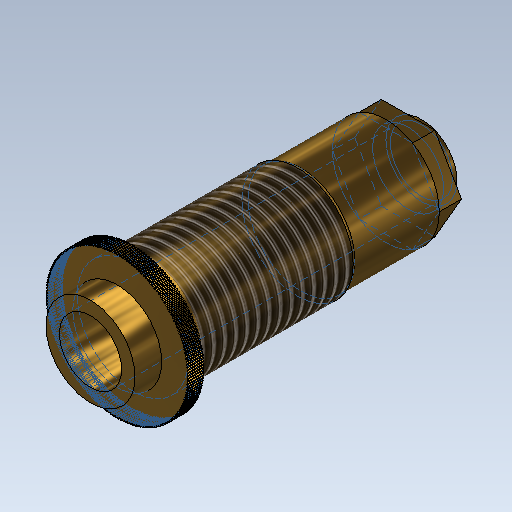
# Autodesk Inventor part: タミヤダンパー2
Saved by Autodesk Inventor 2020 (Build 240168000, 168)
## iProperties
Part Number: タミヤダンパー2
Material: 真鍮
Document SubType Name: Modeling
Designer: 雪村
Density: 8.49 g/cm^3
Appearance: 真鍮 - つや出し
Mass: 24.2679 g
Surface Area: 26.0167 cm^2
Volume: 2.85841 cm^3
Author: 雪村
Autodesk Inventor part; units mm, degrees
(part 1 of 2)
ref_plane "YZ Plane" through (0, 0, 0) normal (1, 0, 0) x (0, 1, 0)
ref_plane "XZ Plane" through (0, 0, 0) normal (0, 1, 0) x (-1, 0, 0)
ref_plane "XY Plane" through (0, 0, 0) normal (0, 0, 1) x (1, 0, 0)
sketch "スケッチ1" plane through (0, 0, 0) normal (0, 0, 1) x (1, 0, 0)
  circle A0 centre (0, 0) radius 5.5
  dimension "d0" = 11
  constraints: 1 centre point, 1 coincident
  measures "d0" diameter of A0
extrude "押し出し1" add sketch "スケッチ1" along normal blind 2.5
sketch "スケッチ2" plane through (0, 0, 2.5) normal (0, 0, 1) x (1, 0, 0)
  circle A0 centre (0, 0) radius 6
  dimension "d3" = 12
  constraints: 1 centre point, 1 coincident
  measures "d3" diameter of A0
extrude "押し出し2" add sketch "スケッチ2" along normal blind 9.5
sketch "スケッチ3" plane through (0, 0, 12) normal (0, 0, 1) x (1, 0, 0)
  circle A0 centre (0, 0) radius 6.25
  dimension "d6" = 12.5
  constraints: 1 centre point, 1 coincident
  measures "d6" diameter of A0
extrude "押し出し3" add sketch "スケッチ3" along normal blind 18.95
sketch "スケッチ4" plane through (0, 0, 30.95) normal (0, 0, 1) x (1, 0, 0)
  circle A0 centre (0, 0) radius 8
  dimension "d9" = 16
  constraints: 1 centre point, 1 coincident
  measures "d9" diameter of A0
extrude "押し出し4" add sketch "スケッチ4" along normal blind 1.75
sketch "スケッチ5" plane through (0, 0, 0) normal (0, 0, -1) x (-1, 0, 0)
  line L0 (-3, -5.1962) -> (-6, 0)
  line L1 (-6, 0) -> (-3, 5.1962)
  line L2 (-3, 5.1962) -> (3, 5.1962)
  line L3 (3, 5.1962) -> (6, 0)
  line L4 (6, 0) -> (3, -5.1962)
  line L5 (3, -5.1962) -> (-3, -5.1962)
  circle A0 centre (0, 0) radius 6 projected
  constraints: 12 end point, 1 coincident, 1 horizontal, 15 other
extrude "押し出し5" add sketch "スケッチ5" against normal blind 2.5 contours L0 L1 L2 L3 L4 L5
sketch "スケッチ6" plane through (0, 0, 0) normal (0, 0, -1) x (-1, 0, 0)
  arc A0 (3.5986, -4.1593) -> (5.4014, -1.0368) centre (0, 0) ccw projected
  line L0 (6, 0) -> (5.4014, -1.0368) projected
  line L1 (5.4014, 1.0368) -> (6, 0) projected
  arc A1 (5.4014, 1.0368) -> (3.5986, 4.1593) centre (0, 0) ccw projected
  line L2 (3, 5.1962) -> (3.5986, 4.1593) projected
  line L3 (1.8028, 5.1962) -> (3, 5.1962) projected
  arc A2 (1.8028, 5.1962) -> (-1.8028, 5.1962) centre (0, 0) ccw projected
  line L4 (-3, 5.1962) -> (-1.8028, 5.1962) projected
  line L5 (-3.5986, 4.1593) -> (-3, 5.1962) projected
  arc A3 (-3.5986, 4.1593) -> (-5.4014, 1.0368) centre (0, 0) ccw projected
  line L6 (-6, 0) -> (-5.4014, 1.0368) projected
  line L7 (-5.4014, -1.0368) -> (-6, 0) projected
  arc A4 (-5.4014, -1.0368) -> (-3.5986, -4.1593) centre (0, 0) ccw projected
  line L8 (-3, -5.1962) -> (-3.5986, -4.1593) projected
  line L9 (-1.8028, -5.1962) -> (-3, -5.1962) projected
  arc A5 (-1.8028, -5.1962) -> (1.8028, -5.1962) centre (0, 0) ccw projected
  line L10 (3, -5.1962) -> (1.8028, -5.1962) projected
  line L11 (3.5986, -4.1593) -> (3, -5.1962) projected
  line L12 (3, -5.1962) -> (-3, -5.1962)
  line L13 (-3, -5.1962) -> (-6, 0)
  line L14 (-6, 0) -> (-3, 5.1962)
  line L15 (-3, 5.1962) -> (3, 5.1962)
  line L16 (3, 5.1962) -> (6, 0)
  line L17 (6, 0) -> (3, -5.1962)
  constraints: 12 end point, 1 coincident, 13 other
extrude "押し出し6" cut sketch "スケッチ6" against normal blind 2.5 contours L17 A0 | A5 L12 | L16 A1 | A4 L13 | L15 A2 | A3 L14
sketch "スケッチ8" plane through (0, 0, 0) normal (0, 0, -1) x (-1, 0, 0)
  circle A0 centre (0, 0) radius 3.5
  dimension "d22" = 7
  constraints: 1 centre point, 1 coincident
  measures "d22" diameter of A0
extrude "押し出し7" cut sketch "スケッチ8" against normal through all
sketch "スケッチ9" plane through (0, 0, 32.7) normal (0, 0, 1) x (1, 0, 0)
  circle A0 centre (0, 0) radius 3.5 projected
  circle A1 centre (0, 0) radius 5
  dimension "d25" = 10
  constraints: 1 centre point, 1 coincident
  measures "d25" diameter of A1
extrude "押し出し8" add sketch "スケッチ9" along normal blind 3
sketch "スケッチ11" plane through (0, 0, 0) normal (0, 0, -1) x (-1, 0, 0)
  circle A0 centre (0, 0) radius 3.5 projected
  circle A1 centre (0, 0) radius 4
  dimension "d28" = 8
  constraints: 1 centre point, 1 coincident
  measures "d28" diameter of A1
extrude "押し出し9" add sketch "スケッチ11" along normal blind 1.5
sketch "スケッチ12" plane through (0, 0, 32.7) normal (0, 0, 1) x (1, 0, 0)
  arc A0 (0.0868, 7.9995) -> (-0.0868, 7.9995) centre (0, 0) ccw
  arc A1 (0.05, 7.8748) -> (-0.05, 7.8748) centre (0, 0) ccw
  line L0 (-0.05, 7.8748) -> (-0.0868, 7.9995)
  line L1 (0.05, 7.8748) -> (0.0868, 7.9995)
  line L2 (0, 7.875) -> (0, 0)
  line L3 (-0.5992, 7.8522) -> (-0.6446, 7.974)
  arc A2 (-0.4714, 7.9861) -> (-0.6446, 7.974) centre (0, 0) ccw
  line L4 (-0.4994, 7.8591) -> (-0.4714, 7.9861)
  arc A3 (-0.4994, 7.8591) -> (-0.5992, 7.8522) centre (0, 0) ccw
  line L5 (-1.1455, 7.7912) -> (-1.1993, 7.9096)
  arc A4 (-1.0274, 7.9338) -> (-1.1993, 7.9096) centre (0, 0) ccw
  line L6 (-1.0465, 7.8052) -> (-1.0274, 7.9338)
  arc A5 (-1.0465, 7.8052) -> (-1.1455, 7.7912) centre (0, 0) ccw
  line L7 (-1.6862, 7.6924) -> (-1.7481, 7.8067)
  arc A6 (-1.5783, 7.8428) -> (-1.7481, 7.8067) centre (0, 0) ccw
  line L8 (-1.5884, 7.7132) -> (-1.5783, 7.8428)
  arc A7 (-1.5884, 7.7132) -> (-1.6862, 7.6924) centre (0, 0) ccw
  line L9 (-2.2187, 7.556) -> (-2.2884, 7.6657)
  arc A8 (-2.1215, 7.7136) -> (-2.2884, 7.6657) centre (0, 0) ccw
  line L10 (-2.1225, 7.5836) -> (-2.1215, 7.7136)
  arc A9 (-2.1225, 7.5836) -> (-2.2187, 7.556) centre (0, 0) ccw
  line L11 (-2.7403, 7.3828) -> (-2.8175, 7.4874)
  arc A10 (-2.6545, 7.5468) -> (-2.8175, 7.4874) centre (0, 0) ccw
  line L12 (-2.6464, 7.417) -> (-2.6545, 7.5468)
  arc A11 (-2.6464, 7.417) -> (-2.7403, 7.3828) centre (0, 0) ccw
  line L13 (-3.2487, 7.1737) -> (-3.333, 7.2726)
  arc A12 (-3.1744, 7.3432) -> (-3.333, 7.2726) centre (0, 0) ccw
  line L14 (-3.1573, 7.2144) -> (-3.1744, 7.3432)
  arc A13 (-3.1573, 7.2144) -> (-3.2487, 7.1737) centre (0, 0) ccw
  line L15 (-3.7412, 6.9296) -> (-3.8322, 7.0224)
  arc A14 (-3.6789, 7.1039) -> (-3.8322, 7.0224) centre (0, 0) ccw
  line L16 (-3.6529, 6.9765) -> (-3.6789, 7.1039)
  arc A15 (-3.6529, 6.9765) -> (-3.7412, 6.9296) centre (0, 0) ccw
  line L17 (-4.2154, 6.6517) -> (-4.3127, 6.738)
  arc A16 (-4.1655, 6.83) -> (-4.3127, 6.738) centre (0, 0) ccw
  line L18 (-4.1306, 6.7047) -> (-4.1655, 6.83)
  arc A17 (-4.1306, 6.7047) -> (-4.2154, 6.6517) centre (0, 0) ccw
  line L19 (-4.6692, 6.3415) -> (-4.7722, 6.4207)
  arc A18 (-4.6318, 6.5228) -> (-4.7722, 6.4207) centre (0, 0) ccw
  line L20 (-4.5883, 6.4003) -> (-4.6318, 6.5228)
  arc A19 (-4.5883, 6.4003) -> (-4.6692, 6.3415) centre (0, 0) ccw
  line L21 (-5.1002, 6.0003) -> (-5.2085, 6.0722)
  arc A20 (-5.0755, 6.1838) -> (-5.2085, 6.0722) centre (0, 0) ccw
  line L22 (-5.0235, 6.0646) -> (-5.0755, 6.1838)
  arc A21 (-5.0235, 6.0646) -> (-5.1002, 6.0003) centre (0, 0) ccw
  line L23 (-5.5063, 5.63) -> (-5.6194, 5.6941)
  arc A22 (-5.4945, 5.8147) -> (-5.6194, 5.6941) centre (0, 0) ccw
  line L24 (-5.4344, 5.6994) -> (-5.4945, 5.8147)
  arc A23 (-5.4344, 5.6994) -> (-5.5063, 5.63) centre (0, 0) ccw
  line L25 (-5.8856, 5.2321) -> (-6.0029, 5.2882)
  arc A24 (-5.8867, 5.4172) -> (-6.0029, 5.2882) centre (0, 0) ccw
  line L26 (-5.8187, 5.3065) -> (-5.8867, 5.4172)
  arc A25 (-5.8187, 5.3065) -> (-5.8856, 5.2321) centre (0, 0) ccw
  line L27 (-6.2362, 4.8088) -> (-6.3571, 4.8566)
  arc A26 (-6.2503, 4.9934) -> (-6.3571, 4.8566) centre (0, 0) ccw
  line L28 (-6.1747, 4.8876) -> (-6.2503, 4.9934)
  arc A27 (-6.1747, 4.8876) -> (-6.2362, 4.8088) centre (0, 0) ccw
  line L29 (-6.5565, 4.3621) -> (-6.6804, 4.4013)
  arc A28 (-6.5834, 4.5452) -> (-6.6804, 4.4013) centre (0, 0) ccw
  line L30 (-6.5006, 4.445) -> (-6.5834, 4.5452)
  arc A29 (-6.5006, 4.445) -> (-6.5565, 4.3621) centre (0, 0) ccw
  line L31 (-6.8448, 3.8941) -> (-6.9712, 3.9246)
  arc A30 (-6.8844, 4.0749) -> (-6.9712, 3.9246) centre (0, 0) ccw
  line L32 (-6.7948, 3.9807) -> (-6.8844, 4.0749)
  arc A31 (-6.7948, 3.9807) -> (-6.8448, 3.8941) centre (0, 0) ccw
  line L33 (-7.0998, 3.4072) -> (-7.228, 3.4288)
  arc A32 (-7.1519, 3.5848) -> (-7.228, 3.4288) centre (0, 0) ccw
  line L34 (-7.0559, 3.497) -> (-7.1519, 3.5848)
  arc A33 (-7.0559, 3.497) -> (-7.0998, 3.4072) centre (0, 0) ccw
  line L35 (-7.3202, 2.9036) -> (-7.4495, 2.9162)
  arc A34 (-7.3845, 3.0771) -> (-7.4495, 2.9162) centre (0, 0) ccw
  line L36 (-7.2827, 2.9963) -> (-7.3845, 3.0771)
  arc A35 (-7.2827, 2.9963) -> (-7.3202, 2.9036) centre (0, 0) ccw
  line L37 (-7.5049, 2.3859) -> (-7.6348, 2.3895)
  arc A36 (-7.5812, 2.5545) -> (-7.6348, 2.3895) centre (0, 0) ccw
  line L38 (-7.474, 2.481) -> (-7.5812, 2.5545)
  arc A37 (-7.474, 2.481) -> (-7.5049, 2.3859) centre (0, 0) ccw
  line L39 (-7.653, 1.8566) -> (-7.7829, 1.8511)
  arc A38 (-7.7409, 2.0195) -> (-7.7829, 1.8511) centre (0, 0) ccw
  line L40 (-7.6288, 1.9536) -> (-7.7409, 2.0195)
  arc A39 (-7.6288, 1.9536) -> (-7.653, 1.8566) centre (0, 0) ccw
  line L41 (-7.7639, 1.3182) -> (-7.8931, 1.3036)
  arc A40 (-7.8629, 1.4746) -> (-7.8931, 1.3036) centre (0, 0) ccw
  line L42 (-7.7465, 1.4167) -> (-7.8629, 1.4746)
  arc A41 (-7.7465, 1.4167) -> (-7.7639, 1.3182) centre (0, 0) ccw
  line L43 (-7.8369, 0.7734) -> (-7.9648, 0.7499)
  arc A42 (-7.9466, 0.9225) -> (-7.9648, 0.7499) centre (0, 0) ccw
  line L44 (-7.8265, 0.8729) -> (-7.9466, 0.9225)
  arc A43 (-7.8265, 0.8729) -> (-7.8369, 0.7734) centre (0, 0) ccw
  line L45 (-7.8718, 0.2249) -> (-7.9977, 0.1925)
  arc A44 (-7.9916, 0.3659) -> (-7.9977, 0.1925) centre (0, 0) ccw
  line L46 (-7.8683, 0.3248) -> (-7.9916, 0.3659)
  arc A45 (-7.8683, 0.3248) -> (-7.8718, 0.2249) centre (0, 0) ccw
  line L47 (-7.8683, -0.3248) -> (-7.9916, -0.3659)
  arc A46 (-7.9977, -0.1925) -> (-7.9916, -0.3659) centre (0, 0) ccw
  line L48 (-7.8718, -0.2249) -> (-7.9977, -0.1925)
  arc A47 (-7.8718, -0.2249) -> (-7.8683, -0.3248) centre (0, 0) ccw
  line L49 (-7.8265, -0.8729) -> (-7.9466, -0.9225)
  arc A48 (-7.9648, -0.7499) -> (-7.9466, -0.9225) centre (0, 0) ccw
  line L50 (-7.8369, -0.7734) -> (-7.9648, -0.7499)
  arc A49 (-7.8369, -0.7734) -> (-7.8265, -0.8729) centre (0, 0) ccw
  line L51 (-7.7465, -1.4167) -> (-7.8629, -1.4746)
  arc A50 (-7.8931, -1.3036) -> (-7.8629, -1.4746) centre (0, 0) ccw
  line L52 (-7.7639, -1.3182) -> (-7.8931, -1.3036)
  arc A51 (-7.7639, -1.3182) -> (-7.7465, -1.4167) centre (0, 0) ccw
  line L53 (-7.6288, -1.9536) -> (-7.7409, -2.0195)
  arc A52 (-7.7829, -1.8511) -> (-7.7409, -2.0195) centre (0, 0) ccw
  line L54 (-7.653, -1.8566) -> (-7.7829, -1.8511)
  arc A53 (-7.653, -1.8566) -> (-7.6288, -1.9536) centre (0, 0) ccw
  line L55 (-7.474, -2.481) -> (-7.5812, -2.5545)
  arc A54 (-7.6348, -2.3895) -> (-7.5812, -2.5545) centre (0, 0) ccw
  line L56 (-7.5049, -2.3859) -> (-7.6348, -2.3895)
  arc A55 (-7.5049, -2.3859) -> (-7.474, -2.481) centre (0, 0) ccw
  line L57 (-7.2827, -2.9963) -> (-7.3845, -3.0771)
  arc A56 (-7.4495, -2.9162) -> (-7.3845, -3.0771) centre (0, 0) ccw
  line L58 (-7.3202, -2.9036) -> (-7.4495, -2.9162)
  arc A57 (-7.3202, -2.9036) -> (-7.2827, -2.9963) centre (0, 0) ccw
  line L59 (-7.0559, -3.497) -> (-7.1519, -3.5848)
  arc A58 (-7.228, -3.4288) -> (-7.1519, -3.5848) centre (0, 0) ccw
  line L60 (-7.0998, -3.4072) -> (-7.228, -3.4288)
  arc A59 (-7.0998, -3.4072) -> (-7.0559, -3.497) centre (0, 0) ccw
  line L61 (-6.7948, -3.9807) -> (-6.8844, -4.0749)
  arc A60 (-6.9712, -3.9246) -> (-6.8844, -4.0749) centre (0, 0) ccw
  line L62 (-6.8448, -3.8941) -> (-6.9712, -3.9246)
  arc A61 (-6.8448, -3.8941) -> (-6.7948, -3.9807) centre (0, 0) ccw
  line L63 (-6.5006, -4.445) -> (-6.5834, -4.5452)
  arc A62 (-6.6804, -4.4013) -> (-6.5834, -4.5452) centre (0, 0) ccw
  line L64 (-6.5565, -4.3621) -> (-6.6804, -4.4013)
  arc A63 (-6.5565, -4.3621) -> (-6.5006, -4.445) centre (0, 0) ccw
  line L65 (-6.1747, -4.8876) -> (-6.2503, -4.9934)
  arc A64 (-6.3571, -4.8566) -> (-6.2503, -4.9934) centre (0, 0) ccw
  line L66 (-6.2362, -4.8088) -> (-6.3571, -4.8566)
  arc A65 (-6.2362, -4.8088) -> (-6.1747, -4.8876) centre (0, 0) ccw
  line L67 (-5.8187, -5.3065) -> (-5.8867, -5.4172)
  arc A66 (-6.0029, -5.2882) -> (-5.8867, -5.4172) centre (0, 0) ccw
  line L68 (-5.8856, -5.2321) -> (-6.0029, -5.2882)
  arc A67 (-5.8856, -5.2321) -> (-5.8187, -5.3065) centre (0, 0) ccw
  line L69 (-5.4344, -5.6994) -> (-5.4945, -5.8147)
  arc A68 (-5.6194, -5.6941) -> (-5.4945, -5.8147) centre (0, 0) ccw
  line L70 (-5.5063, -5.63) -> (-5.6194, -5.6941)
  arc A69 (-5.5063, -5.63) -> (-5.4344, -5.6994) centre (0, 0) ccw
  line L71 (-5.0235, -6.0646) -> (-5.0755, -6.1838)
  arc A70 (-5.2085, -6.0722) -> (-5.0755, -6.1838) centre (0, 0) ccw
  line L72 (-5.1002, -6.0003) -> (-5.2085, -6.0722)
  arc A71 (-5.1002, -6.0003) -> (-5.0235, -6.0646) centre (0, 0) ccw
  line L73 (-4.5883, -6.4003) -> (-4.6318, -6.5228)
  arc A72 (-4.7722, -6.4207) -> (-4.6318, -6.5228) centre (0, 0) ccw
  line L74 (-4.6692, -6.3415) -> (-4.7722, -6.4207)
  arc A73 (-4.6692, -6.3415) -> (-4.5883, -6.4003) centre (0, 0) ccw
  line L75 (-4.1306, -6.7047) -> (-4.1655, -6.83)
  arc A74 (-4.3127, -6.738) -> (-4.1655, -6.83) centre (0, 0) ccw
  line L76 (-4.2154, -6.6517) -> (-4.3127, -6.738)
  arc A75 (-4.2154, -6.6517) -> (-4.1306, -6.7047) centre (0, 0) ccw
  line L77 (-3.6529, -6.9765) -> (-3.6789, -7.1039)
  arc A76 (-3.8322, -7.0224) -> (-3.6789, -7.1039) centre (0, 0) ccw
  line L78 (-3.7412, -6.9296) -> (-3.8322, -7.0224)
  arc A77 (-3.7412, -6.9296) -> (-3.6529, -6.9765) centre (0, 0) ccw
  line L79 (-3.1573, -7.2144) -> (-3.1744, -7.3432)
  arc A78 (-3.333, -7.2726) -> (-3.1744, -7.3432) centre (0, 0) ccw
  line L80 (-3.2487, -7.1737) -> (-3.333, -7.2726)
  arc A79 (-3.2487, -7.1737) -> (-3.1573, -7.2144) centre (0, 0) ccw
  line L81 (-2.6464, -7.417) -> (-2.6545, -7.5468)
  arc A80 (-2.8175, -7.4874) -> (-2.6545, -7.5468) centre (0, 0) ccw
  line L82 (-2.7403, -7.3828) -> (-2.8175, -7.4874)
  arc A81 (-2.7403, -7.3828) -> (-2.6464, -7.417) centre (0, 0) ccw
  line L83 (-2.1225, -7.5836) -> (-2.1215, -7.7136)
  arc A82 (-2.2884, -7.6657) -> (-2.1215, -7.7136) centre (0, 0) ccw
  line L84 (-2.2187, -7.556) -> (-2.2884, -7.6657)
  arc A83 (-2.2187, -7.556) -> (-2.1225, -7.5836) centre (0, 0) ccw
  line L85 (-1.5884, -7.7132) -> (-1.5783, -7.8428)
  arc A84 (-1.7481, -7.8067) -> (-1.5783, -7.8428) centre (0, 0) ccw
  line L86 (-1.6862, -7.6924) -> (-1.7481, -7.8067)
  arc A85 (-1.6862, -7.6924) -> (-1.5884, -7.7132) centre (0, 0) ccw
  line L87 (-1.0465, -7.8052) -> (-1.0274, -7.9338)
  arc A86 (-1.1993, -7.9096) -> (-1.0274, -7.9338) centre (0, 0) ccw
  line L88 (-1.1455, -7.7912) -> (-1.1993, -7.9096)
  arc A87 (-1.1455, -7.7912) -> (-1.0465, -7.8052) centre (0, 0) ccw
  line L89 (-0.4994, -7.8591) -> (-0.4714, -7.9861)
  arc A88 (-0.6446, -7.974) -> (-0.4714, -7.9861) centre (0, 0) ccw
  line L90 (-0.5992, -7.8522) -> (-0.6446, -7.974)
  arc A89 (-0.5992, -7.8522) -> (-0.4994, -7.8591) centre (0, 0) ccw
  line L91 (0.05, -7.8748) -> (0.0868, -7.9995)
  arc A90 (-0.0868, -7.9995) -> (0.0868, -7.9995) centre (0, 0) ccw
  line L92 (-0.05, -7.8748) -> (-0.0868, -7.9995)
  arc A91 (-0.05, -7.8748) -> (0.05, -7.8748) centre (0, 0) ccw
  line L93 (0.5992, -7.8522) -> (0.6446, -7.974)
  arc A92 (0.4714, -7.9861) -> (0.6446, -7.974) centre (0, 0) ccw
  line L94 (0.4994, -7.8591) -> (0.4714, -7.9861)
  arc A93 (0.4994, -7.8591) -> (0.5992, -7.8522) centre (0, 0) ccw
  line L95 (1.1455, -7.7912) -> (1.1993, -7.9096)
  arc A94 (1.0274, -7.9338) -> (1.1993, -7.9096) centre (0, 0) ccw
  line L96 (1.0465, -7.8052) -> (1.0274, -7.9338)
  arc A95 (1.0465, -7.8052) -> (1.1455, -7.7912) centre (0, 0) ccw
  line L97 (1.6862, -7.6924) -> (1.7481, -7.8067)
  arc A96 (1.5783, -7.8428) -> (1.7481, -7.8067) centre (0, 0) ccw
  line L98 (1.5884, -7.7132) -> (1.5783, -7.8428)
  arc A97 (1.5884, -7.7132) -> (1.6862, -7.6924) centre (0, 0) ccw
  line L99 (2.2187, -7.556) -> (2.2884, -7.6657)
  arc A98 (2.1215, -7.7136) -> (2.2884, -7.6657) centre (0, 0) ccw
  line L100 (2.1225, -7.5836) -> (2.1215, -7.7136)
  arc A99 (2.1225, -7.5836) -> (2.2187, -7.556) centre (0, 0) ccw
  line L101 (2.7403, -7.3828) -> (2.8175, -7.4874)
  arc A100 (2.6545, -7.5468) -> (2.8175, -7.4874) centre (0, 0) ccw
  line L102 (2.6464, -7.417) -> (2.6545, -7.5468)
  arc A101 (2.6464, -7.417) -> (2.7403, -7.3828) centre (0, 0) ccw
  line L103 (3.2487, -7.1737) -> (3.333, -7.2726)
  arc A102 (3.1744, -7.3432) -> (3.333, -7.2726) centre (0, 0) ccw
  line L104 (3.1573, -7.2144) -> (3.1744, -7.3432)
  arc A103 (3.1573, -7.2144) -> (3.2487, -7.1737) centre (0, 0) ccw
  line L105 (3.7412, -6.9296) -> (3.8322, -7.0224)
  arc A104 (3.6789, -7.1039) -> (3.8322, -7.0224) centre (0, 0) ccw
  line L106 (3.6529, -6.9765) -> (3.6789, -7.1039)
  arc A105 (3.6529, -6.9765) -> (3.7412, -6.9296) centre (0, 0) ccw
  line L107 (4.2154, -6.6517) -> (4.3127, -6.738)
  arc A106 (4.1655, -6.83) -> (4.3127, -6.738) centre (0, 0) ccw
  line L108 (4.1306, -6.7047) -> (4.1655, -6.83)
  arc A107 (4.1306, -6.7047) -> (4.2154, -6.6517) centre (0, 0) ccw
  line L109 (4.6692, -6.3415) -> (4.7722, -6.4207)
  arc A108 (4.6318, -6.5228) -> (4.7722, -6.4207) centre (0, 0) ccw
  line L110 (4.5883, -6.4003) -> (4.6318, -6.5228)
  arc A109 (4.5883, -6.4003) -> (4.6692, -6.3415) centre (0, 0) ccw
  line L111 (5.1002, -6.0003) -> (5.2085, -6.0722)
  arc A110 (5.0755, -6.1838) -> (5.2085, -6.0722) centre (0, 0) ccw
  line L112 (5.0235, -6.0646) -> (5.0755, -6.1838)
  arc A111 (5.0235, -6.0646) -> (5.1002, -6.0003) centre (0, 0) ccw
  line L113 (5.5063, -5.63) -> (5.6194, -5.6941)
  arc A112 (5.4945, -5.8147) -> (5.6194, -5.6941) centre (0, 0) ccw
  line L114 (5.4344, -5.6994) -> (5.4945, -5.8147)
  arc A113 (5.4344, -5.6994) -> (5.5063, -5.63) centre (0, 0) ccw
  line L115 (5.8856, -5.2321) -> (6.0029, -5.2882)
  arc A114 (5.8867, -5.4172) -> (6.0029, -5.2882) centre (0, 0) ccw
  line L116 (5.8187, -5.3065) -> (5.8867, -5.4172)
  arc A115 (5.8187, -5.3065) -> (5.8856, -5.2321) centre (0, 0) ccw
  line L117 (6.2362, -4.8088) -> (6.3571, -4.8566)
  arc A116 (6.2503, -4.9934) -> (6.3571, -4.8566) centre (0, 0) ccw
  line L118 (6.1747, -4.8876) -> (6.2503, -4.9934)
  arc A117 (6.1747, -4.8876) -> (6.2362, -4.8088) centre (0, 0) ccw
  line L119 (6.5565, -4.3621) -> (6.6804, -4.4013)
  arc A118 (6.5834, -4.5452) -> (6.6804, -4.4013) centre (0, 0) ccw
  line L120 (6.5006, -4.445) -> (6.5834, -4.5452)
  arc A119 (6.5006, -4.445) -> (6.5565, -4.3621) centre (0, 0) ccw
  line L121 (6.8448, -3.8941) -> (6.9712, -3.9246)
  arc A120 (6.8844, -4.0749) -> (6.9712, -3.9246) centre (0, 0) ccw
  line L122 (6.7948, -3.9807) -> (6.8844, -4.0749)
  arc A121 (6.7948, -3.9807) -> (6.8448, -3.8941) centre (0, 0) ccw
  line L123 (7.0998, -3.4072) -> (7.228, -3.4288)
  arc A122 (7.1519, -3.5848) -> (7.228, -3.4288) centre (0, 0) ccw
  line L124 (7.0559, -3.497) -> (7.1519, -3.5848)
  arc A123 (7.0559, -3.497) -> (7.0998, -3.4072) centre (0, 0) ccw
  line L125 (7.3202, -2.9036) -> (7.4495, -2.9162)
  arc A124 (7.3845, -3.0771) -> (7.4495, -2.9162) centre (0, 0) ccw
  line L126 (7.2827, -2.9963) -> (7.3845, -3.0771)
  arc A125 (7.2827, -2.9963) -> (7.3202, -2.9036) centre (0, 0) ccw
  line L127 (7.5049, -2.3859) -> (7.6348, -2.3895)
  arc A126 (7.5812, -2.5545) -> (7.6348, -2.3895) centre (0, 0) ccw
  line L128 (7.474, -2.481) -> (7.5812, -2.5545)
  arc A127 (7.474, -2.481) -> (7.5049, -2.3859) centre (0, 0) ccw
  line L129 (7.653, -1.8566) -> (7.7829, -1.8511)
  arc A128 (7.7409, -2.0195) -> (7.7829, -1.8511) centre (0, 0) ccw
  line L130 (7.6288, -1.9536) -> (7.7409, -2.0195)
  arc A129 (7.6288, -1.9536) -> (7.653, -1.8566) centre (0, 0) ccw
  line L131 (7.7639, -1.3182) -> (7.8931, -1.3036)
  arc A130 (7.8629, -1.4746) -> (7.8931, -1.3036) centre (0, 0) ccw
  line L132 (7.7465, -1.4167) -> (7.8629, -1.4746)
  arc A131 (7.7465, -1.4167) -> (7.7639, -1.3182) centre (0, 0) ccw
  line L133 (7.8369, -0.7734) -> (7.9648, -0.7499)
  arc A132 (7.9466, -0.9225) -> (7.9648, -0.7499) centre (0, 0) ccw
  line L134 (7.8265, -0.8729) -> (7.9466, -0.9225)
  arc A133 (7.8265, -0.8729) -> (7.8369, -0.7734) centre (0, 0) ccw
  line L135 (7.8718, -0.2249) -> (7.9977, -0.1925)
  arc A134 (7.9916, -0.3659) -> (7.9977, -0.1925) centre (0, 0) ccw
  line L136 (7.8683, -0.3248) -> (7.9916, -0.3659)
  arc A135 (7.8683, -0.3248) -> (7.8718, -0.2249) centre (0, 0) ccw
  line L137 (7.8683, 0.3248) -> (7.9916, 0.3659)
  arc A136 (7.9977, 0.1925) -> (7.9916, 0.3659) centre (0, 0) ccw
  line L138 (7.8718, 0.2249) -> (7.9977, 0.1925)
  arc A137 (7.8718, 0.2249) -> (7.8683, 0.3248) centre (0, 0) ccw
  line L139 (7.8265, 0.8729) -> (7.9466, 0.9225)
  arc A138 (7.9648, 0.7499) -> (7.9466, 0.9225) centre (0, 0) ccw
  line L140 (7.8369, 0.7734) -> (7.9648, 0.7499)
  arc A139 (7.8369, 0.7734) -> (7.8265, 0.8729) centre (0, 0) ccw
  line L141 (7.7465, 1.4167) -> (7.8629, 1.4746)
  arc A140 (7.8931, 1.3036) -> (7.8629, 1.4746) centre (0, 0) ccw
  line L142 (7.7639, 1.3182) -> (7.8931, 1.3036)
  arc A141 (7.7639, 1.3182) -> (7.7465, 1.4167) centre (0, 0) ccw
  line L143 (7.6288, 1.9536) -> (7.7409, 2.0195)
  arc A142 (7.7829, 1.8511) -> (7.7409, 2.0195) centre (0, 0) ccw
  line L144 (7.653, 1.8566) -> (7.7829, 1.8511)
  arc A143 (7.653, 1.8566) -> (7.6288, 1.9536) centre (0, 0) ccw
  line L145 (7.474, 2.481) -> (7.5812, 2.5545)
  arc A144 (7.6348, 2.3895) -> (7.5812, 2.5545) centre (0, 0) ccw
  line L146 (7.5049, 2.3859) -> (7.6348, 2.3895)
  arc A145 (7.5049, 2.3859) -> (7.474, 2.481) centre (0, 0) ccw
  line L147 (7.2827, 2.9963) -> (7.3845, 3.0771)
  arc A146 (7.4495, 2.9162) -> (7.3845, 3.0771) centre (0, 0) ccw
  line L148 (7.3202, 2.9036) -> (7.4495, 2.9162)
  arc A147 (7.3202, 2.9036) -> (7.2827, 2.9963) centre (0, 0) ccw
  line L149 (7.0559, 3.497) -> (7.1519, 3.5848)
  arc A148 (7.228, 3.4288) -> (7.1519, 3.5848) centre (0, 0) ccw
  line L150 (7.0998, 3.4072) -> (7.228, 3.4288)
  arc A149 (7.0998, 3.4072) -> (7.0559, 3.497) centre (0, 0) ccw
  line L151 (6.7948, 3.9807) -> (6.8844, 4.0749)
  arc A150 (6.9712, 3.9246) -> (6.8844, 4.0749) centre (0, 0) ccw
  line L152 (6.8448, 3.8941) -> (6.9712, 3.9246)
  arc A151 (6.8448, 3.8941) -> (6.7948, 3.9807) centre (0, 0) ccw
  line L153 (6.5006, 4.445) -> (6.5834, 4.5452)
  arc A152 (6.6804, 4.4013) -> (6.5834, 4.5452) centre (0, 0) ccw
  line L154 (6.5565, 4.3621) -> (6.6804, 4.4013)
  arc A153 (6.5565, 4.3621) -> (6.5006, 4.445) centre (0, 0) ccw
  line L155 (6.1747, 4.8876) -> (6.2503, 4.9934)
  arc A154 (6.3571, 4.8566) -> (6.2503, 4.9934) centre (0, 0) ccw
  line L156 (6.2362, 4.8088) -> (6.3571, 4.8566)
  arc A155 (6.2362, 4.8088) -> (6.1747, 4.8876) centre (0, 0) ccw
  line L157 (5.8187, 5.3065) -> (5.8867, 5.4172)
  arc A156 (6.0029, 5.2882) -> (5.8867, 5.4172) centre (0, 0) ccw
  line L158 (5.8856, 5.2321) -> (6.0029, 5.2882)
  arc A157 (5.8856, 5.2321) -> (5.8187, 5.3065) centre (0, 0) ccw
  line L159 (5.4344, 5.6994) -> (5.4945, 5.8147)
  arc A158 (5.6194, 5.6941) -> (5.4945, 5.8147) centre (0, 0) ccw
  line L160 (5.5063, 5.63) -> (5.6194, 5.6941)
  arc A159 (5.5063, 5.63) -> (5.4344, 5.6994) centre (0, 0) ccw
  line L161 (5.0235, 6.0646) -> (5.0755, 6.1838)
  arc A160 (5.2085, 6.0722) -> (5.0755, 6.1838) centre (0, 0) ccw
  line L162 (5.1002, 6.0003) -> (5.2085, 6.0722)
  arc A161 (5.1002, 6.0003) -> (5.0235, 6.0646) centre (0, 0) ccw
  line L163 (4.5883, 6.4003) -> (4.6318, 6.5228)
  arc A162 (4.7722, 6.4207) -> (4.6318, 6.5228) centre (0, 0) ccw
  line L164 (4.6692, 6.3415) -> (4.7722, 6.4207)
  arc A163 (4.6692, 6.3415) -> (4.5883, 6.4003) centre (0, 0) ccw
  line L165 (4.1306, 6.7047) -> (4.1655, 6.83)
  arc A164 (4.3127, 6.738) -> (4.1655, 6.83) centre (0, 0) ccw
  line L166 (4.2154, 6.6517) -> (4.3127, 6.738)
  arc A165 (4.2154, 6.6517) -> (4.1306, 6.7047) centre (0, 0) ccw
  line L167 (3.6529, 6.9765) -> (3.6789, 7.1039)
  arc A166 (3.8322, 7.0224) -> (3.6789, 7.1039) centre (0, 0) ccw
  line L168 (3.7412, 6.9296) -> (3.8322, 7.0224)
  arc A167 (3.7412, 6.9296) -> (3.6529, 6.9765) centre (0, 0) ccw
  line L169 (3.1573, 7.2144) -> (3.1744, 7.3432)
  arc A168 (3.333, 7.2726) -> (3.1744, 7.3432) centre (0, 0) ccw
  line L170 (3.2487, 7.1737) -> (3.333, 7.2726)
  arc A169 (3.2487, 7.1737) -> (3.1573, 7.2144) centre (0, 0) ccw
  line L171 (2.6464, 7.417) -> (2.6545, 7.5468)
  arc A170 (2.8175, 7.4874) -> (2.6545, 7.5468) centre (0, 0) ccw
  line L172 (2.7403, 7.3828) -> (2.8175, 7.4874)
  arc A171 (2.7403, 7.3828) -> (2.6464, 7.417) centre (0, 0) ccw
  line L173 (2.1225, 7.5836) -> (2.1215, 7.7136)
  arc A172 (2.2884, 7.6657) -> (2.1215, 7.7136) centre (0, 0) ccw
  line L174 (2.2187, 7.556) -> (2.2884, 7.6657)
  arc A173 (2.2187, 7.556) -> (2.1225, 7.5836) centre (0, 0) ccw
  line L175 (1.5884, 7.7132) -> (1.5783, 7.8428)
  arc A174 (1.7481, 7.8067) -> (1.5783, 7.8428) centre (0, 0) ccw
  line L176 (1.6862, 7.6924) -> (1.7481, 7.8067)
  arc A175 (1.6862, 7.6924) -> (1.5884, 7.7132) centre (0, 0) ccw
  line L177 (1.0465, 7.8052) -> (1.0274, 7.9338)
  arc A176 (1.1993, 7.9096) -> (1.0274, 7.9338) centre (0, 0) ccw
  line L178 (1.1455, 7.7912) -> (1.1993, 7.9096)
  arc A177 (1.1455, 7.7912) -> (1.0465, 7.8052) centre (0, 0) ccw
  line L179 (0.4994, 7.8591) -> (0.4714, 7.9861)
  arc A178 (0.6446, 7.974) -> (0.4714, 7.9861) centre (0, 0) ccw
  line L180 (0.5992, 7.8522) -> (0.6446, 7.974)
  arc A179 (0.5992, 7.8522) -> (0.4994, 7.8591) centre (0, 0) ccw
  point P0 (-0.5493, 7.8558)
  point P1 (-1.096, 7.7984)
  point P2 (-1.6373, 7.7029)
  point P3 (-2.1706, 7.5699)
  point P4 (-2.6934, 7.4001)
  point P5 (-3.2031, 7.1942)
  point P6 (-3.6971, 6.9532)
  point P7 (-4.1731, 6.6784)
  point P8 (-4.6288, 6.371)
  point P9 (-5.062, 6.0326)
  point P10 (-5.4704, 5.6648)
  point P11 (-5.8523, 5.2694)
  point P12 (-6.2056, 4.8483)
  point P13 (-6.5287, 4.4036)
  point P14 (-6.82, 3.9375)
  point P15 (-7.078, 3.4522)
  point P16 (-7.3016, 2.95)
  point P17 (-7.4896, 2.4335)
  point P18 (-7.6411, 1.9051)
  point P19 (-7.7554, 1.3675)
  point P20 (-7.8319, 0.8232)
  point P21 (-7.8702, 0.2748)
  point P22 (-7.8702, -0.2748)
  point P23 (-7.8319, -0.8232)
  point P24 (-7.7554, -1.3675)
  point P25 (-7.6411, -1.9051)
  point P26 (-7.4896, -2.4335)
  point P27 (-7.3016, -2.95)
  point P28 (-7.078, -3.4522)
  point P29 (-6.82, -3.9375)
  point P30 (-6.5287, -4.4036)
  point P31 (-6.2056, -4.8483)
  point P32 (-5.8523, -5.2694)
  point P33 (-5.4704, -5.6648)
  point P34 (-5.062, -6.0326)
  point P35 (-4.6288, -6.371)
  point P36 (-4.1731, -6.6784)
  point P37 (-3.6971, -6.9532)
  point P38 (-3.2031, -7.1942)
  point P39 (-2.6934, -7.4001)
  point P40 (-2.1706, -7.5699)
  point P41 (-1.6373, -7.7029)
  point P42 (-1.096, -7.7984)
  point P43 (-0.5493, -7.8558)
  point P44 (0, -7.875)
  point P45 (0.5493, -7.8558)
  point P46 (1.096, -7.7984)
  point P47 (1.6373, -7.7029)
  point P48 (2.1706, -7.5699)
  point P49 (2.6934, -7.4001)
  point P50 (3.2031, -7.1942)
  point P51 (3.6971, -6.9532)
  point P52 (4.1731, -6.6784)
  point P53 (4.6288, -6.371)
  point P54 (5.062, -6.0326)
  point P55 (5.4704, -5.6648)
  point P56 (5.8523, -5.2694)
  point P57 (6.2056, -4.8483)
  point P58 (6.5287, -4.4036)
  point P59 (6.82, -3.9375)
  point P60 (7.078, -3.4522)
  point P61 (7.3016, -2.95)
  point P62 (7.4896, -2.4335)
  point P63 (7.6411, -1.9051)
  point P64 (7.7554, -1.3675)
  point P65 (7.8319, -0.8232)
  point P66 (7.8702, -0.2748)
  point P67 (7.8702, 0.2748)
  point P68 (7.8319, 0.8232)
  point P69 (7.7554, 1.3675)
  point P70 (7.6411, 1.9051)
  point P71 (7.4896, 2.4335)
  point P72 (7.3016, 2.95)
  point P73 (7.078, 3.4522)
  point P74 (6.82, 3.9375)
  point P75 (6.5287, 4.4036)
  point P76 (6.2056, 4.8483)
  point P77 (5.8523, 5.2694)
  point P78 (5.4704, 5.6648)
  point P79 (5.062, 6.0326)
  point P80 (4.6288, 6.371)
  point P81 (4.1731, 6.6784)
  point P82 (3.6971, 6.9532)
  point P83 (3.2031, 7.1942)
  point P84 (2.6934, 7.4001)
  point P85 (2.1706, 7.5699)
  point P86 (1.6373, 7.7029)
  point P87 (1.096, 7.7984)
  point P88 (0.5493, 7.8558)
  dimension "d31" = 15.75
  dimension "d33" = 0.13
  dimension "d34" = 0.13
  dimension "d35" = 0.1
  dimension "d36" = 0.05
  dimension "d39" = 360
  constraints: 450 point on circle, 362 end point, 180 centre point, 90 coincident, 1 vertical, 992 other
  measures "d31" diameter of A1
  measures "d33" distance of L0.start L0.end
  measures "d34" distance of L1.start L1.end
  measures "d35" distance of L1.start L0.start
  measures "d36" distance from line of L2 L0.start
extrude "押し出し11" cut sketch "スケッチ12" against normal through all